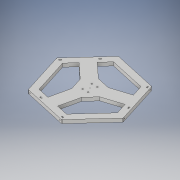
# Autodesk Inventor part: Hex_Servo_Top
Saved by Autodesk Inventor 2019 (Build 230136000, 136)
## iProperties
Created: 2019-09-26
Part Number: Hex_Servo_Top
Material: Generic
Document SubType Name: Modeling
Designer: Jorian Bruslind
Density: 1 g/cm^3
Appearance: Default
Author: Jorian Bruslind
Autodesk Inventor part; units mm, degrees
ref_plane "YZ Plane" through (0, 0, 0) normal (1, 0, 0) x (0, 1, 0)
ref_plane "XZ Plane" through (0, 0, 0) normal (0, 1, 0) x (-1, 0, 0)
ref_plane "XY Plane" through (0, 0, 0) normal (0, 0, 1) x (1, 0, 0)
sketch "Sketch1" plane through (0, 0, 0) normal (0, 1, 0) x (-1, 0, 0)
  line L0 (67.5641, 73.7231) -> (97.6281, -21.6506)
  line L1 (97.6281, -21.6506) -> (30.0641, -95.3738)
  line L2 (30.0641, -95.3738) -> (-67.5641, -73.7231)
  line L3 (-67.5641, -73.7231) -> (-97.6281, 21.6506)
  line L4 (-97.6281, 21.6506) -> (-30.0641, 95.3738)
  line L5 (-30.0641, 95.3738) -> (67.5641, 73.7231)
  point P0 (0, 0)
  point P1 (0, 0)
  dimension "d0" = 100
  dimension "d17" = 21.6506
  constraints: 12 end point, 1 coincident, 13 other
  measures "d0" distance of L0.end L1.end
  measures "d17" vertical distance of L4.end L0.start
extrude "Extrusion1" add sketch "Sketch1" along normal blind 8
sketch "Sketch2" plane through (67.5641, 0, -73.7231) normal (0.9537375, 0, -0.3006406) x (-0.3006406, 0, -0.9537375)
  line L0 (0, 0) -> (0, 8) projected
  line L1 (0, 4) -> (-5, 4)
  line L2 (-100, 0) -> (-100, 8) projected
  line L3 (-100, 4) -> (-95, 4)
  circle A0 centre (-95, 4) radius 1
  circle A1 centre (-5, 4) radius 1
  point P0 (-50, 0)
  dimension "d4" = 5
  dimension "d5" = 5
  dimension "d6" = 2
  dimension "d7" = 2
  constraints: 4 end point, 2 centre point, 2 coincident, 2 horizontal, 2 midpoint
  measures "d4" distance of L1.start L1.end
  measures "d5" distance of L3.start L3.end
  measures "d6" diameter of A0
  measures "d7" diameter of A1
extrude "Extrusion2" cut sketch "Sketch2" against normal blind 10
sketch "Sketch3" plane through (0, 8, 0) normal (0, 1, 0) x (1, 0, 0)
  circle A0 centre (0, 0) radius 0.5
  dimension "d10" = 1
  constraints: 1 centre point, 1 coincident
  measures "d10" diameter of A0
extrude "Extrusion3" cut sketch "Sketch3" against normal blind 5
pattern_circular "Circular Pattern1" count 3 over 360 about axis through (0, 8, 0) along (0, -1, 0) of "Extrusion2"
sketch "Sketch4" plane through (0, 8, 0) normal (0, 1, 0) x (1, 0, 0)
  line L0 (0, 0) -> (0, 10.5)
  line L1 (0, 10.5) -> (-6.25, 10.5)
  circle A0 centre (-6.25, 10.5) radius 1.5
  circle A1 centre (6.25, 10.5) radius 1.5
  circle A2 centre (-6.25, -10.5) radius 1.5
  circle A3 centre (6.25, -10.5) radius 1.5
  dimension "d18" = 10.5
  dimension "d19" = 6.25
  dimension "d20" = 3
  dimension "d23" = 12.5
  dimension "d26" = 21
  constraints: 4 centre point, 4 end point, 2 vertical, 1 coincident, 1 horizontal, 1 perpendicular, 6 other
  measures "d18" distance of L0.start L0.end
  measures "d19" distance of L0.end L1.end
  measures "d20" diameter of A0
  measures "d23" distance of A0.centre A1.centre
  measures "d26" distance of A0.centre A2.centre
extrude "Extrusion4" cut sketch "Sketch4" against normal blind 8
sketch "Sketch5" plane through (0, 8, 0) normal (0, 1, 0) x (1, 0, 0)
  line L0 (-67.5641, -73.7231) -> (30.0641, -95.3738) projected
  line L1 (30.0641, -95.3738) -> (25.1827, -94.2912)
  line L2 (25.1827, -94.2912) -> (26.0487, -90.3861)
  line L3 (26.0487, -90.3861) -> (23.9985, -89.9314)
  line L4 (26.0487, -90.3861) -> (28.0989, -90.8408)
  line L5 (23.9985, -89.9314) -> (24.5398, -87.4907)
  line L6 (24.5398, -87.4907) -> (28.6401, -88.4001)
  line L7 (28.6401, -88.4001) -> (28.0989, -90.8408)
  point P0 (0, 0)
  dimension "d31" = 5
  dimension "d32" = 4
  dimension "d33" = 2.1
  dimension "d34" = 90
  dimension "d35" = 2.1
  dimension "d36" = 90
  dimension "d37" = 2.5
  dimension "d38" = 90
  dimension "d39" = 90
  constraints: 14 end point, 2 perpendicular, 1 point on line
  measures "d31" distance of L0.end L1.end
  measures "d32" distance of L1.end L2.end
  measures "d33" distance of L2.end L3.end
  measures "d34" angle of L3 L2
  measures "d35" distance of L2.end L4.end
  measures "d36" angle of L2 L4
  measures "d37" distance of L3.end L5.end
  measures "d38" angle of L3 L5
  measures "d39" angle of L5 L6
extrude "Extrusion5" cut sketch "Sketch5" against normal blind 8
pattern_linear "Rectangular Pattern1" count 2 spacing 65 along (-0.9762812, 0, -0.2165064) of "Extrusion5"
pattern_circular "Circular Pattern2" count 3 over 360 about axis through (0, 8, 0) along (0, -1, 0) of "Extrusion5", "Rectangular Pattern1"
sketch "Sketch6" plane through (0, 8, 0) normal (0, 1, 0) x (1, 0, 0)
  line L0 (-97.6281, 21.6506) -> (-30.0641, 95.3738) projected
  line L1 (-97.6281, 21.6506) -> (-30.0641, 95.3738)
  line L2 (-30.0641, 95.3738) -> (67.5641, 73.7231) projected
  line L3 (-30.0641, 95.3738) -> (67.5641, 73.7231)
  line L4 (67.5641, 73.7231) -> (97.6281, -21.6506) projected
  line L5 (67.5641, 73.7231) -> (97.6281, -21.6506)
  line L6 (97.6281, -21.6506) -> (30.0641, -95.3738) projected
  line L7 (97.6281, -21.6506) -> (30.0641, -95.3738)
  line L8 (30.0641, -95.3738) -> (-67.5641, -73.7231)
  line L9 (-61.7064, -75.0222) -> (-63.6589, -74.5891) projected
  line L10 (-67.5641, -73.7231) -> (-97.6281, 21.6506)
  line L11 (-80.7184, 17.9006) -> (-24.8568, 78.8545)
  line L12 (-24.8568, 78.8545) -> (55.8616, 60.9539)
  line L13 (55.8616, 60.9539) -> (80.7184, -17.9006)
  line L14 (80.7184, -17.9006) -> (24.8568, -78.8545)
  line L15 (24.8568, -78.8545) -> (-55.8616, -60.9539)
  line L16 (-55.8616, -60.9539) -> (-80.7184, 17.9006)
  line L17 (0, 0) -> (30, 0) construction
  line L18 (8.8449, -28.0592) -> (28.7224, -6.3697)
  line L19 (28.7224, -6.3697) -> (19.8775, 21.6895)
  line L20 (19.8775, 21.6895) -> (-8.8449, 28.0592)
  line L21 (-8.8449, 28.0592) -> (-28.7224, 6.3697)
  line L22 (-28.7224, 6.3697) -> (-19.8775, -21.6895)
  line L23 (-19.8775, -21.6895) -> (8.8449, -28.0592)
  line L24 (28.7224, -6.3697) -> (19.8775, 21.6895)
  line L25 (-8.8449, 28.0592) -> (-28.7224, 6.3697)
  line L26 (-19.8775, -21.6895) -> (8.8449, -28.0592)
  line L27 (0, 0) -> (8.8449, -28.0592)
  line L28 (-8.8449, 28.0592) -> (-28.7224, 6.3697)
  line L29 (-28.7224, 6.3697) -> (-62.7264, 37.5328)
  line L30 (-62.7264, 37.5328) -> (-42.8489, 59.2223)
  line L31 (-42.8489, 59.2223) -> (-8.8449, 28.0592)
  line L32 (-19.8775, -21.6895) -> (8.8449, -28.0592)
  line L33 (8.8449, -28.0592) -> (-1.1412, -73.089)
  line L34 (-1.1412, -73.089) -> (-29.8636, -66.7194)
  line L35 (-29.8636, -66.7194) -> (-19.8775, -21.6895)
  line L36 (28.7224, -6.3697) -> (19.8775, 21.6895)
  line L37 (19.8775, 21.6895) -> (63.8676, 35.5562)
  line L38 (63.8676, 35.5562) -> (72.7125, 7.497)
  line L39 (72.7125, 7.497) -> (28.7224, -6.3697)
  dimension "d50" = 15
  dimension "d53" = 28.7224
  constraints: 70 end point, 10 collinear, 9 parallel, 3 perpendicular, 1 horizontal, 10 other
  measures "d50" distance between parallel lines of L10 L16
  measures "d53" horizontal distance of L19.end L20.end
fillet "Fillet2" radius 2 6 edges at (-97.6281, 4, -21.6506) (-67.5641, 4, 73.7231) (30.0641, 4, 95.3738) (97.6281, 4, 21.6506) (67.5641, 4, -73.7231) (-30.0641, 4, -95.3738)
extrude "Extrusion7" cut sketch "Sketch6" against normal blind 10 contours L11 L29 L22 L35 L15 L16 | L11 L12 L13 L37 L20 L31 | L33 L18 L39 L13 L14 L15
body "Solid1"
